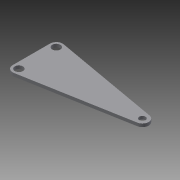
# Autodesk Inventor part: x_axis_shaft_support
Saved by Autodesk Inventor 2013 (Build 170138000, 138)
## iProperties
Created: 2013-09-17
Part Number: x_axis_shaft_support
Material: Generic
Document SubType Name: Modeling
Designer: Ian
Density: 1 g/cm^3
Mass: 11.5457 g
Surface Area: 84.3819 cm^2
Volume: 11.5457 cm^3
Author: Ian
Autodesk Inventor part; units mm, degrees
ref_plane "YZ Plane" through (0, 0, 0) normal (1, 0, 0) x (0, 1, 0)
ref_plane "XZ Plane" through (0, 0, 0) normal (0, 1, 0) x (-1, 0, 0)
ref_plane "XY Plane" through (0, 0, 0) normal (0, 0, 1) x (1, 0, 0)
sketch "Sketch1" plane through (0, 0, 0) normal (0, 1, 0) x (-1, 0, 0)
  circle A0 centre (0, 19.05) radius 4.1656
  circle A1 centre (0, -19.05) radius 4.1656
  circle A2 centre (-106.68, 0) radius 3.175
  arc A3 (6.35, 19.05) -> (-1.1163, 25.3011) centre (0, 19.05) ccw
  arc A4 (-1.1163, -25.3011) -> (6.35, -19.05) centre (0, -19.05) ccw
  line L0 (0, 19.05) -> (-106.68, 0) construction
  line L1 (-106.68, 0) -> (0, -19.05) construction
  line L2 (-107.7963, -6.2511) -> (-1.1163, -25.3011)
  line L3 (-107.7963, 6.2511) -> (-1.1163, 25.3011)
  line L4 (-132.5233, 0) -> (35.4452, 0) construction
  line L5 (6.35, 19.05) -> (6.35, -19.05)
  arc A5 (-107.7963, 6.2511) -> (-107.7963, -6.2511) centre (-106.68, 0) ccw
  point P0 (0, 0)
  dimension "d0" = 38.1
  dimension "d2" = 19.05
  dimension "d3" = 106.68
  dimension "d4" = 8.3312
  dimension "d5" = 8.3312
  dimension "d6" = 6.35
  dimension "d8" = 12.7
  dimension "d9" = 12.7
  dimension "d10" = 20.249
  dimension "d11" = 6.35
  dimension "d12" = 79.875
  dimension "d13" = 0
  dimension "d14" = 29.0952
  dimension "d15" = 138.8733
  constraints: 12 end point, 7 point on circle, 6 centre point, 6 coincident, 5 tangent, 1 horizontal, 1 parallel, 1 point on line, 1 vertical
  measures "d0" distance of point (0, -19.05) point (0, 19.05)
  measures "d2" distance of point (0, 0) point (0, 19.05)
  measures "d3" distance of point (0, 0) point (-106.68, 0)
  measures "d4" diameter of A0
  measures "d5" diameter of A1
  measures "d6" diameter of A2
  measures "d8" diameter of A3
  measures "d9" diameter of A4
  measures "d10" angle of L0 L1
  measures "d11" radius of A5
  measures "d12" angle of L5 L0
  measures "d13" distance from line of point (0, 0) L4
  measures "d14" distance from line of L4.end L5
  measures "d15" distance from line of L4.start L5
extrude "Extrusion1" add sketch "Sketch1" along normal blind 3.175
equation "\"d2\" = 0.5 * d0"
equation "\"d5\" = d4"
body "Solid1"
